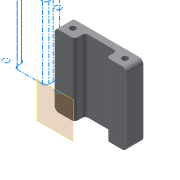
# Autodesk Inventor part: 10_Base_v0_plate
Saved by Autodesk Inventor 2019.4 (Build 234330000, 330)
## iProperties
Created: 2020-05-27
Part Number: 10_Base_v0_plate
Material: Generic
Document SubType Name: Modeling
Designer: diederichbenedict
Density: 1 g/cm^3
Appearance: Default
Author: diederichbenedict
Autodesk Inventor part; units mm, degrees
ref_plane "YZ Plane" through (0, 0, 0) normal (1, 0, 0) x (0, 1, 0)
ref_plane "XZ Plane" through (0, 0, 0) normal (0, 1, 0) x (-1, 0, 0)
ref_plane "Work Plane1" through (0, 0, 0) normal (0, 0, 1) x (1, 0, 0)
sketch "Sketch1" plane through (0, 0, 0) normal (0, 0, 1) x (1, 0, 0)
  line L0 (9.1, -25) -> (9.1, -17.5) projected
  line L1 (9.1, -25) -> (25, -25) projected
  line L2 (25, -25) -> (25, -9.1) projected
  line L3 (17.5, -9.1) -> (25, -9.1) projected
  line L4 (17.5, -9.1) -> (17.5, -15.5) projected
  arc A0 (15.5, -17.5) -> (17.5, -15.5) centre (15.5, -15.5) ccw projected
  line L5 (15.5, -17.5) -> (9.1, -17.5) projected
  circle A1 centre (20, -20) radius 2.2989 projected
  arc A2 (17.5, 15.5) -> (15.5, 17.5) centre (15.5, 15.5) ccw projected
  line L6 (-15.25, 17.25) -> (15.25, 17.25)
  line L7 (17.25, 15.25) -> (17.25, -15.25)
  line L8 (15.25, -17.25) -> (-15.25, -17.25)
  line L9 (-17.25, -15.25) -> (-17.25, 15.25)
  line L10 (-17.25, 17.25) -> (17.25, -17.25) construction
  line L11 (17.25, 17.25) -> (-17.25, -17.25) construction
  arc A3 (15.25, -17.25) -> (17.25, -15.25) centre (15.25, -15.25) ccw
  arc A4 (-17.25, -15.25) -> (-15.25, -17.25) centre (-15.25, -15.25) ccw
  arc A5 (-15.25, 17.25) -> (-17.25, 15.25) centre (-15.25, 15.25) ccw
  arc A6 (17.25, 15.25) -> (15.25, 17.25) centre (15.25, 15.25) ccw
  point P0 (0, 0)
  dimension "d0" = 34.5
  dimension "d1" = 34.5
  dimension "d2" = 2
  constraints: 12 end point, 8 point on circle, 8 point on line, 8 tangent, 4 centre point, 3 equal radius, 2 midpoint, 2 parallel, 1 horizontal, 1 perpendicular
  measures "d0" distance of L10.end L11.end
  measures "d1" distance of L11.start L10.end
  measures "d2" radius of A3
ref_plane "Work Plane2" through (-25, -25, -8) normal (0, 0, -1) x (0, 1, 0)
extrude "Extrusion1" add sketch "Sketch1" against normal up to surface (8 mm away) contours L6 A6 L7 A3 L8 A4 L9 A5
sketch "Sketch2" plane through (-15.25, 17.25, 0) normal (0, 1, 0) x (1, 0, 0)
  arc A0 (22.85, 1.5) -> (24.35, 0) centre (24.35, 1.5) ccw projected
  line L0 (40.25, 0) -> (24.35, 0) projected
  line L1 (40.25, 0) -> (40.25, 8) projected
  line L2 (18.4, 8) -> (40.25, 8) projected
  line L3 (18.4, 8) -> (18.4, 5) projected
  line L4 (18.4, 5) -> (21.35, 5) projected
  arc A1 (22.85, 3.5) -> (21.35, 5) centre (21.35, 3.5) ccw projected
  line L5 (22.85, 3.5) -> (22.85, 1.5) projected
  circle A2 centre (27.75, 4) radius 1.75 projected
  circle A3 centre (2.75, 4) radius 1.75 projected
  arc A4 (6.15, 0) -> (7.65, 1.5) centre (6.15, 1.5) ccw projected
  line L6 (7.65, 1.5) -> (7.65, 3.5) projected
  arc A5 (9.15, 5) -> (7.65, 3.5) centre (9.15, 3.5) ccw projected
  line L7 (9.15, 5) -> (12.1, 5) projected
  line L8 (12.1, 5) -> (12.1, 8) projected
  line L9 (-9.75, 8) -> (12.1, 8) projected
  line L10 (-9.75, 0) -> (-9.75, 8) projected
  line L11 (6.15, 0) -> (-9.75, 0) projected
  line L12 (18.4, 5) -> (12.1, 5)
  line L13 (12.1, 5) -> (12.1, 8)
  line L14 (12.1, 8) -> (18.4, 8)
  line L15 (18.4, 8) -> (18.4, 5)
  line L16 (24.35, 0) -> (6.15, 0)
  circle A6 centre (27.75, 4) radius 1.4
  circle A7 centre (2.75, 4) radius 1.4
  point P0 (15.25, 0)
  dimension "d7" = 2.8
  dimension "d8" = 2.8
  constraints: 10 end point, 2 centre point, 2 coincident, 2 parallel, 1 collinear, 1 horizontal, 1 perpendicular, 1 tangent
  measures "d7" diameter of A6
  measures "d8" diameter of A7
extrude "Extrusion2" cut sketch "Sketch2" against normal through all contours A0 L16 A4 L6 A5 L7 L12 L4 A1 L5 | A6 | A7
sketch "Sketch3" plane through (-6.1, 17.25, -5) normal (0, 0, 1) x (1, 0, 0)
  circle A0 centre (6.1, -17.25) radius 4.7436
  constraints: 1 centre point, 1 coincident
pattern_circular "Circular Pattern1" count 2 over 90 about axis through (0, 0, -5) along (0, 0, 1) of "Extrusion2"
body "Solid1"
